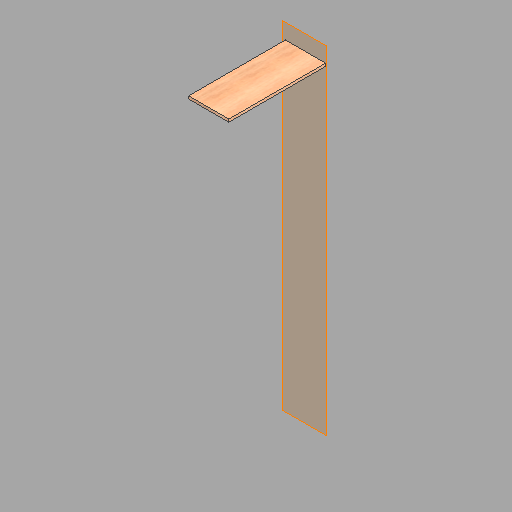
# Autodesk Inventor part: SH2.1
Saved by Autodesk Inventor 2025.2 (Build 292293000, 293)
## iProperties
Created: 2025-01-27
Part Number: SH2.1
Material: Wood (Birch)
Document SubType Name: Modeling
Designer: Anna
Density: 0.55 g/cm^3
Appearance: Birch - Natural Polished
Mass: 1970.44 g
Surface Area: 4124.19 cm^2
Volume: 3582.62 cm^3
Author: Anna
Autodesk Inventor part; units mm, degrees
ref_plane "Work Plane1" through (-15.8748, 0, 0) normal (0, 0, 1) x (1, 0, 0)
sketch "Sketch1" plane through (-15.8748, 0, 0) normal (0, 0, 1) x (1, 0, 0)
  line L0 (147.6374, 1066.8) -> (147.6374, 1047.75)
  line L1 (147.6374, 1047.75) -> (-131.7626, 1047.75)
  line L2 (-131.7626, 1047.75) -> (-131.7626, 1066.8)
  line L3 (-131.7626, 1066.8) -> (147.6374, 1066.8)
  point P0 (15.8748, 0)
  point P1 (147.6374, 1057.275)
  point P2 (-131.7626, 1057.275)
  dimension "d0" = 19.05
  dimension "d3" = 279.4
  constraints: 8 end point, 2 midpoint, 2 perpendicular, 1 horizontal, 1 vertical
  measures "d0" distance of L0.start L0.end
  measures "d3" distance of point (147.637, 1057.275) point (-131.763, 1057.275)
ref_plane "Work Plane2" through (-139.7, -1066.8, 927.1) normal (0, 0, -1) x (0, 1, 0)
ref_plane "Work Plane3" through (-147.6374, -1066.8, 933.45) normal (0, 0, -1) x (0, 1, 0)
ref_plane "Work Plane4" through (-147.6374, -1066.8, 939.8) normal (0, 0, -1) x (0, 1, 0)
ref_plane "Work Plane5" through (-147.6374, 159.15, 673.1) normal (0, 0, -1) x (0, 1, 0)
extrude "Extrusion1" add sketch "Sketch1" along normal up to surface (673.1 mm away)
body "Solid1"
